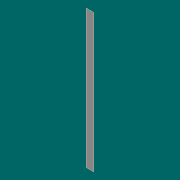
# Autodesk Inventor part: coluredSpacer
Saved by Autodesk Inventor 2016 SP1 (Build 200210100, 210)
## iProperties
Created: 2016-02-15
Part Number: coluredSpacer
Material: ABS Plastic
Document SubType Name: Modeling
Designer: sawai
Density: 1.06 g/cm^3
Appearance: Smooth - White
Author: sawai
Autodesk Inventor part; units mm, degrees
ref_plane "YZ Plane" through (0, 0, 0) normal (1, 0, 0) x (0, 1, 0)
ref_plane "XZ Plane" through (0, 0, 0) normal (0, 1, 0) x (-1, 0, 0)
ref_plane "XY Plane" through (0, 0, 0) normal (0, 0, 1) x (1, 0, 0)
sketch "Sketch1" plane through (0, 0, 0) normal (0, 1, 0) x (-1, 0, 0)
  line L0 (-5.7, 100.35) -> (5.7, 100.35)
  line L1 (5.7, 100.35) -> (5.7, -100.35)
  line L2 (5.7, -100.35) -> (-5.7, -100.35)
  line L3 (-5.7, -100.35) -> (-5.7, 100.35)
  line L4 (-5.7, 100.35) -> (5.7, -100.35) construction
  line L5 (5.7, 100.35) -> (-5.7, -100.35) construction
  point P0 (0, 0)
  dimension "d0" = 11.4
  dimension "d1" = 200.7
  constraints: 12 end point, 2 midpoint, 2 parallel, 1 horizontal, 1 perpendicular
  measures "d0" distance of L1.end L2.end
  measures "d1" distance of L2.end L0.start
extrude "Extrusion1" add sketch "Sketch1" along normal blind 0.1
equation "\"d0\" = 2 * rubberizedCoating + ScintillatorThickness + 2 * silveringThickness"
equation "\"d1\" = silveringThickness + ScintillatorHeight + rubberizedCoating"
equation "\"OpticalFiberDiameter\" = 1"
equation "\"OpticalFiberClearence\" = 0.1"
equation "\"ScintillatorEdgeClearence\" = 3"
equation "\"ScintillatorWidth\" = 25"
equation "\"ScintillatorHeight\" = 200"
equation "\"ShallowTrackDepth\" = 1.2"
equation "\"DeepTrackDepth\" = 5.6"
equation "\"FiberEdgeOffsett\" = 5"
equation "\"LoopLargeTrackRatio\" = 1.1"
equation "\"FiberSensorClerence\" = 0.5"
equation "\"MountingScrewOffsett\" = 9"
equation "\"silveringThickness\" = 0.2"
equation "\"rubberizedCoating\" = 0.5"
equation "\"ScintillatorThickness\" = 10"
body "Solid1"
